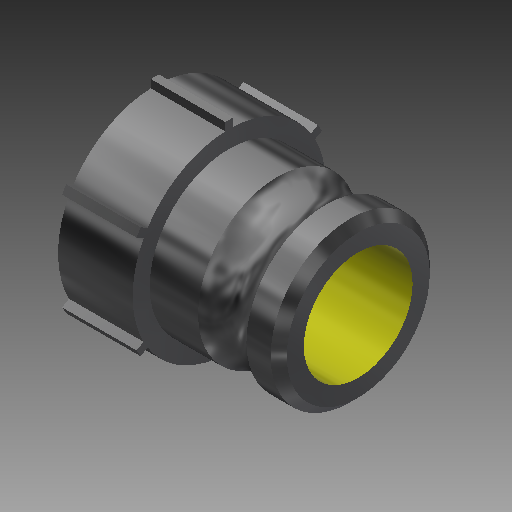
# Autodesk Inventor part: banjo female cam
Saved by Autodesk Inventor 2017 (Build 210142000, 142)
## iProperties
Created: 2014-07-07
Part Number: banjo female cam
Material: GFRP
Description: Cam Lock, 2" SS-Male Adapter x Female NPT, (BANJO P/N 200A)
Document SubType Name: Modeling
Designer: mrister
Engineer: mrister
Density: 1.75 g/cm^3
Appearance: Rubber - Black - Version 1.1
Author: mrister
Autodesk Inventor part; units mm, degrees
ref_plane "YZ Plane" through (0, 0, 0) normal (1, 0, 0) x (0, 1, 0)
ref_plane "XZ Plane" through (0, 0, 0) normal (0, 1, 0) x (-1, 0, 0)
ref_plane "XY Plane" through (0, 0, 0) normal (0, 0, 1) x (1, 0, 0)
sketch "Sketch1" plane through (0, 0, 0) normal (0, 0, 1) x (1, 0, 0)
  line L0 (3.9687, 31.3531) -> (23.0187, 31.3531)
  line L1 (0, 21.4312) -> (54.7687, 21.4313)
  line L2 (54.7687, 21.4313) -> (54.7687, 28.1781)
  line L3 (54.7687, 28.1781) -> (51.5938, 31.3531)
  line L4 (51.5938, 31.3531) -> (42.0688, 31.3531)
  arc A0 (23.0187, 31.3531) -> (42.0688, 31.3531) centre (32.5437, 46.2926) ccw
  line L5 (-41.4338, 0) -> (70.8025, 0) projected
  line L6 (3.9687, 31.3531) -> (3.9687, 38.1)
  line L7 (3.9687, 38.1) -> (-25.4, 38.1)
  line L8 (-25.4, 38.1) -> (-25.4, 28.575)
  line L9 (-25.4, 28.575) -> (0, 28.575)
  line L10 (0, 28.575) -> (0, 21.4312)
  line L11 (0, 21.4312) -> (0, 0) construction
  point P0 (32.5437, 28.575)
  dimension "d2" = 31.3531
  dimension "d3" = 45
  dimension "d5" = 12.7
  dimension "d6" = 19.05
  dimension "d8" = 28.575
  dimension "d9" = 3.175
  dimension "d27" = 21.4312
  dimension "d28" = 38.1
  dimension "d29" = 29.3687
  dimension "d30" = 50.8
  dimension "d31" = 25.4
  dimension "d32" = 28.575
  constraints: 22 end point, 4 parallel, 3 point on circle, 2 perpendicular, 1 centre point, 1 collinear, 1 horizontal, 1 vertical
  measures "d2" distance from line of L11.end L0
  measures "d3" angle of L2 L3
  measures "d5" distance from line of L4.end L2
  measures "d6" distance of L0.start L0.end
  measures "d8" vertical distance of L11.end point (32.544, 28.575)
  measures "d9" distance from line of L2 L3.end
  measures "d27" distance from line of L11.end L1
  measures "d28" distance from line of L11.end L7
  measures "d29" distance of L6.end L7.end
  measures "d30" distance between parallel lines of L2 L6
  measures "d31" distance of L8.end L9.end
  measures "d32" distance from line of L11.end L9
revolve "Revolution1" add sketch "Sketch1" angle 360 about axis through (-10, 0, 0) along (1, 0, 0)
sketch "Sketch4" plane through (-25.4, 0, 0) normal (-1, 0, 0) x (0, 0, 1)
  circle A0 centre (0, 0) radius 38.1 projected
  circle A1 centre (0, 0) radius 28.575 projected
  line L0 (-1.5875, 41.2419) -> (1.5875, 41.2419)
  line L1 (1.5875, 41.2419) -> (1.5875, 38.0669)
  line L2 (1.5875, 38.0669) -> (-1.5875, 38.0669)
  line L3 (-1.5875, 38.0669) -> (-1.5875, 41.2419)
  line L4 (0, 38.0669) -> (0, 0) construction
  line L5 (-36.5103, 19.2461) -> (-34.9228, 21.9958)
  line L6 (-34.9228, 21.9958) -> (-32.1732, 20.4083)
  line L7 (-32.1732, 20.4083) -> (-33.7607, 17.6586)
  line L8 (-33.7607, 17.6586) -> (-36.5103, 19.2461)
  line L9 (-32.9669, 19.0335) -> (0, 0) construction
  line L10 (36.5103, 19.2461) -> (34.9228, 21.9958)
  line L11 (34.9228, 21.9958) -> (32.1732, 20.4083)
  line L12 (32.1732, 20.4083) -> (33.7607, 17.6586)
  line L13 (33.7607, 17.6586) -> (36.5103, 19.2461)
  line L14 (0, 0) -> (-38.1, 0) construction
  line L15 (-1.5875, -41.2419) -> (1.5875, -41.2419)
  line L16 (1.5875, -41.2419) -> (1.5875, -38.0669)
  line L17 (1.5875, -38.0669) -> (-1.5875, -38.0669)
  line L18 (-1.5875, -38.0669) -> (-1.5875, -41.2419)
  line L19 (-36.5103, -19.2461) -> (-34.9228, -21.9958)
  line L20 (-34.9228, -21.9958) -> (-32.1732, -20.4083)
  line L21 (-32.1732, -20.4083) -> (-33.7607, -17.6586)
  line L22 (-33.7607, -17.6586) -> (-36.5103, -19.2461)
  line L23 (32.1732, -20.4083) -> (33.7607, -17.6586)
  line L24 (33.7607, -17.6586) -> (36.5103, -19.2461)
  line L25 (34.9228, -21.9958) -> (32.1732, -20.4083)
  line L26 (36.5103, -19.2461) -> (34.9228, -21.9958)
  dimension "d33" = 3.175
  dimension "d35" = 60
  constraints: 54 end point, 16 symmetric about line, 5 equal length, 4 parallel, 4 perpendicular, 3 point on circle, 2 midpoint, 1 horizontal
  measures "d33" distance of L0.start L0.end
  measures "d35" angle of L4 L9
extrude "Extrusion3" add sketch "Sketch4" against normal blind 29.3688 contours L12 A0 | A0 L11 L10 L13 | L24 L26 L25 A0 | A0 L23 | L2 A0 | A0 L3 L0 L1 | L16 L15 L18 A0 | A0 L17 | L7 A0 | A0 L8 L5 L6 | L20 L19 L22 A0 | A0 L21
sketch "Sketch5" plane through (0, 0, 0) normal (0, 0, 1) x (1, 0, 0)
  line L0 (0, 28.575) -> (-25.4, 28.575) projected
  line L1 (-28.8575, 28.575) -> (-28.0637, 28.575)
  line L2 (-28.0637, 28.575) -> (-28.4606, 29.3687)
  line L3 (-28.4606, 29.3687) -> (-28.8575, 28.575)
  line L4 (-28.4606, 29.3687) -> (-28.4606, 28.575) construction
  point P0 (0, 0)
  dimension "d40" = 0.7937
  dimension "d42" = 0.7937
  constraints: 8 end point, 2 collinear, 1 midpoint, 1 vertical
  measures "d40" distance of L1.start L1.end
  measures "d42" distance of L2.end L4.end
coil "Coil1" sketch "Sketch5" operation cut axis through (-10, 0, 0) along (1, 0, 0) pitch 1.0583 turns 30 hand right
equation "\"d42\" = d40"
body "Solid1"
